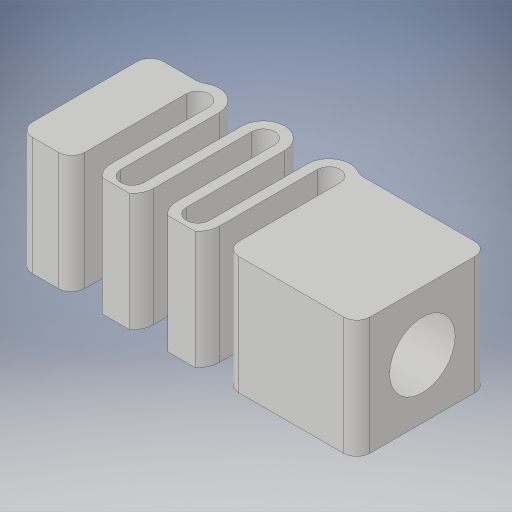
# Autodesk Inventor part: BT505_trajan20_22
Saved by Autodesk Inventor 2023 (Build 270158000, 158)
## iProperties
Company: HTBLA Kaindorf
RuleStatus: InUse
Created: 2022-11-29
Part Number: BT505_trajan20_22
Project: Zeichenmaschine_neu
Material: Generisch
Description: Stifthalterung_3DDruck
Document SubType Name: Modeling
Designer: trajan20
Density: 1 g/cm^3
Appearance: Vorgabe
Mass: 9.79969 g
Surface Area: 72.4575 cm^2
Volume: 9.79969 cm^3
AfterDocNew0: iProperties-Editor_aufrufen
Author: jan
Keywords: 2022
Autodesk Inventor part; units mm, degrees
note: some values were not read from the file. Chosen so that the rebuilt part matches the saved one: direction of "Bohrung1".
ref_plane "YZ Plane" through (0, 0, 0) normal (1, 0, 0) x (0, 1, 0)
ref_plane "XZ Plane" through (0, 0, 0) normal (0, 1, 0) x (-1, 0, 0)
ref_plane "XY Plane" through (0, 0, 0) normal (0, 0, 1) x (1, 0, 0)
sketch "Skizze3" plane through (0, 0, 0) normal (0, 0, 1) x (1, 0, 0)
  line L0 (0, 0) -> (0, 8)
  line L1 (0, 8) -> (20, 8)
  line L2 (20, 0) -> (0, 0)
  arc A0 (2.5, 22.25) -> (2.5, 17.25) centre (2.5, 19.75) ccw construction
  arc A1 (17.5, 12.25) -> (17.5, 17.25) centre (17.5, 14.75) ccw construction
  line L3 (17.5, 17.25) -> (2.5, 17.25) construction
  line L4 (2.5, 22.25) -> (17.5, 22.25) construction
  arc A2 (17.5, 22.25) -> (17.5, 27.25) centre (17.5, 24.75) ccw construction
  arc A3 (4.4592, 31.3029) -> (2.5, 27.25) centre (2.5, 29.75) ccw construction
  line L5 (17.5, 27.25) -> (2.5, 27.25) construction
  line L6 (2.5, 12.25) -> (17.5, 12.25) construction
  arc A4 (2.5, 12.25) -> (0.7146, 8) centre (2.5, 9.75) ccw construction
  line L7 (0, 31.5) -> (0, 51.5)
  line L8 (0, 51.5) -> (20, 51.5)
  arc A5 (0, 31.8267) -> (2.5, 26.5) centre (2.5, 29.75) ccw
  line L9 (2.5, 26.5) -> (17.5, 26.5)
  arc A6 (17.5, 23) -> (17.5, 26.5) centre (17.5, 24.75) ccw
  line L10 (17.5, 23) -> (2.5, 23)
  arc A7 (2.5, 23) -> (2.5, 16.5) centre (2.5, 19.75) ccw
  line L11 (2.5, 16.5) -> (17.5, 16.5)
  arc A8 (17.5, 13) -> (17.5, 16.5) centre (17.5, 14.75) ccw
  line L12 (17.5, 13) -> (2.5, 13)
  arc A9 (2.5, 13) -> (0, 7.6733) centre (2.5, 9.75) ccw
  arc A10 (2.5, 31.5) -> (2.5, 28) centre (2.5, 29.75) ccw
  line L13 (2.5, 28) -> (17.5, 28)
  arc A11 (17.5, 21.5) -> (17.5, 28) centre (17.5, 24.75) ccw
  line L14 (17.5, 21.5) -> (2.5, 21.5)
  arc A12 (2.5, 21.5) -> (2.5, 18) centre (2.5, 19.75) ccw
  line L15 (2.5, 18) -> (17.5, 18)
  arc A13 (17.5, 11.5) -> (17.5, 18) centre (17.5, 14.75) ccw
  line L16 (17.5, 11.5) -> (2.5, 11.5)
  arc A14 (2.5, 11.5) -> (2.5, 8) centre (2.5, 9.75) ccw
  line L17 (0, 31.5) -> (20, 31.5)
  line L18 (20, 31.5) -> (20, 31.5)
  line L19 (20, 31.5) -> (20, 41.5)
  line L20 (20, 51.5) -> (20, 41.5)
  line L21 (20, 31.5) -> (45, 31.5)
  line L22 (45, 31.5) -> (45, 41.5)
  line L23 (45, 41.5) -> (20, 41.5)
  line L24 (20, 0) -> (20, 8)
  point P0 (10, 4)
  point P1 (0, 4)
  point P2 (10, 0)
  dimension "d4" = 8
  dimension "d11" = 5
  dimension "d12" = 5
  dimension "d13" = 5
  dimension "d14" = 5
  dimension "d17" = 5
  dimension "d19" = 0.75
  dimension "d20" = 0.75
  dimension "d22" = 20
  dimension "d23" = 20
  dimension "d24" = 10
  dimension "d29" = 25
  dimension "d54" = 20
  constraints: 51 end point, 30 point on circle, 15 centre point, 15 tangent, 6 horizontal, 6 point on line, 5 perpendicular, 2 midpoint, 2 parallel, 2 vertical, 1 collinear, 1 horizontal alignment, 1 vertical alignment, 16 other
  measures "d4" distance between parallel lines of L2 L1
  measures "d11" diameter of A1
  measures "d12" diameter of A0
  measures "d13" diameter of A2
  measures "d14" diameter of A3
  measures "d17" diameter of A4
  measures "d19" distance between parallel lines of L6 L12
  measures "d20" distance between parallel lines of L6 L16
  measures "d22" distance between parallel lines of L8 L17
  measures "d23" distance between parallel lines of L7 L19
  measures "d24" distance of L18.end L19.end
  measures "d29" distance between parallel lines of L19 L22
  measures "d54" distance between parallel lines of L0 L24
extrude "Extrusion3" add sketch "Skizze3" along normal blind 18
sketch "Skizze4" plane through (20, 31.5, 0) normal (0, 1, 0) x (1, 0, 0)
  circle A0 centre (16, -9) radius 2
  line L0 (25, 0) -> (25, -18) projected
  line L1 (25, -18) -> (0, -18) projected
  line L2 (25, 0) -> (0, 0) projected
  circle A1 centre (6, -9) radius 2.5
  line L3 (0, 0) -> (0, -18) projected
  arc A2 (16, -18) -> (16, 0) centre (16, -9) ccw
  line L4 (0, -18) -> (25, -18) projected
  arc A3 (16, 0) -> (16, -18) centre (16, -9) ccw construction
  circle A4 centre (6, -9) radius 5.25
  point P0 (25, -9)
  point P1 (25, -9)
  point P2 (21, -1.5167)
  dimension "d31" = 4
  dimension "d36" = 5
  dimension "d37" = 6
  dimension "d38" = 10
  dimension "d57" = 10.5
  constraints: 5 centre point, 4 point on circle, 2 coincident, 2 horizontal alignment, 2 point on line, 1 midpoint, 1 tangent
  measures "d31" diameter of A0
  measures "d36" diameter of A1
  measures "d37" distance from line of L3 A1.centre
  measures "d38" distance of A1.centre A0.centre
  measures "d57" diameter of A4
sketch "Skizze6" plane through (0, 51.5, 0) normal (0, 1, 0) x (1, 0, 0)
  circle A0 centre (10, -9) radius 5
  line L0 (20, -18) -> (0, -18) projected
  line L1 (0, 0) -> (0, -18) projected
  point P0 (10, -18)
  point P1 (0, -9)
  dimension "d51" = 10
  constraints: 2 midpoint, 1 centre point, 1 horizontal alignment, 1 vertical alignment
  measures "d51" diameter of A0
extrude "Extrusion9" cut sketch "Skizze6" against normal through all
extrude "Extrusion6" cut sketch "Skizze4" along normal blind 18 contours L0 A2 L2 | L0 L1 A2 | A1
extrude "Extrusion7" add sketch "Skizze4" against normal blind 10 contours A0
hole "Bohrung1" at (10, 4, 0) direction (0, 0, 1) diameter 2.459 end up to surface thread size "M3x0.5" class "6H" standard "ISO Metric profile"
fillet "Rundung3" radius 2 8 edges at (0, 51.5, 9) (20, 51.5, 9) (20, 41.5, 9) (20, 0, 9) (20, 8, 9) (0, 0, 9) (0, 7.6733, 9) (0, 31.8267, 9)
sketch "Skizze7" plane through (0, 0, 18) normal (0, 0, 1) x (1, 0, 0)
  line L0 (20, 43.5) -> (20, 49.5) projected
  line L1 (20, 43.5) -> (50, 43.5)
  line L2 (50, 43.5) -> (50, 0)
  line L3 (50, 0) -> (20, 0)
  line L4 (20, 0) -> (20, 43.5)
  line L5 (2, 0) -> (18, 0) projected
  point P0 (0, 0)
  point P1 (35, 0)
  dimension "d68" = 30
  constraints: 8 end point, 2 parallel, 1 horizontal, 1 midpoint, 1 perpendicular, 1 point on line
  measures "d68" distance between parallel lines of L4 L2
extrude "Extrusion11" cut sketch "Skizze7" against normal through all
fillet "Rundung4" radius 2 1 edges at (20, 31.5, 9)
equation "\"d12\" = d11"
